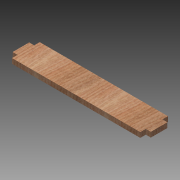
# Autodesk Inventor part: vigas
Saved by Autodesk Inventor 2016 (Build 200138000, 138)
## iProperties
Created: 2016-03-02
Part Number: vigas
Material: Wood (Birch)
Document SubType Name: Modeling
Designer: iberopuebla
Density: 0.55 g/cm^3
Appearance: Birch - Natural Polished
Author: iberopuebla
Autodesk Inventor part; units mm, degrees
ref_plane "YZ Plane" through (0, 0, 0) normal (1, 0, 0) x (0, 1, 0)
ref_plane "XZ Plane" through (0, 0, 0) normal (0, 1, 0) x (-1, 0, 0)
ref_plane "XY Plane" through (0, 0, 0) normal (0, 0, 1) x (1, 0, 0)
sketch "Sketch1" plane through (0, 0, 0) normal (0, 0, 1) x (1, 0, 0)
  line L0 (393.6245, -95.4118) -> (-70.3755, -95.4118)
  line L1 (-70.3755, 4.5882) -> (17.6245, 4.5882)
  line L2 (117.6245, 4.5882) -> (205.6245, 4.5882)
  line L3 (305.6245, 4.5882) -> (393.6245, 4.5882)
  line L4 (-88.3755, -15.4118) -> (-70.3755, -15.4118)
  line L5 (-70.3755, -75.4118) -> (-88.3755, -75.4118)
  line L6 (-88.3755, -75.4118) -> (-88.3755, -15.4118)
  line L7 (-70.3755, -95.4118) -> (-70.3755, -75.4118)
  line L8 (-70.3755, -15.4118) -> (-70.3755, 4.5882)
  line L9 (393.6245, -15.4118) -> (411.6245, -15.4118)
  line L10 (411.6245, -15.4118) -> (411.6245, -75.4118)
  line L11 (411.6245, -75.4118) -> (393.6245, -75.4118)
  line L12 (393.6245, 4.5882) -> (393.6245, -15.4118)
  line L13 (393.6245, -75.4118) -> (393.6245, -95.4118)
  line L14 (17.6245, 4.5882) -> (117.6245, 4.5882)
  line L15 (205.6245, 4.5882) -> (305.6245, 4.5882)
  point P0 (0, 0)
  dimension "d0" = 464
  dimension "d4" = 100
  dimension "d9" = 100
  dimension "d13" = 18
  dimension "d14" = 60
  dimension "d17" = 20
  dimension "d19" = 60
  dimension "d20" = 18
  dimension "d21" = 100
  constraints: 32 end point, 9 parallel, 7 perpendicular, 6 horizontal, 1 collinear
  measures "d0" distance of L0.start L0.end
  measures "d4" distance of L2.start L1.end
  measures "d9" distance of L3.start L2.end
  measures "d13" distance of L5.start L5.end
  measures "d14" distance of L4.end L5.start
  measures "d17" distance between parallel lines of L0 L5
  measures "d19" distance between parallel lines of L11 L9
  measures "d20" distance of L9.start L9.end
  measures "d21" distance between parallel lines of L0 L3
extrude "Extrusion1" add sketch "Sketch1" along normal blind 18
sketch "Sketch3" plane through (0, 0, 18) normal (0, 0, 1) x (1, 0, 0)
  line L0 (-70.3755, -15.4118) -> (-71.5069, -14.2805)
  line L1 (-70.3755, -15.4118) -> (-68.7755, -15.4118) construction
  line L2 (-70.3755, -75.4118) -> (-71.5069, -76.5432)
  line L3 (393.6245, -15.4118) -> (394.7558, -14.2805)
  line L4 (393.6245, -75.4118) -> (394.7558, -76.5432)
  circle A0 centre (-71.5069, -14.2805) radius 1.6
  circle A1 centre (-71.5069, -76.5432) radius 1.6
  circle A2 centre (394.7558, -14.2805) radius 1.6
  circle A3 centre (394.7558, -76.5432) radius 1.6
  point P0 (0, 0)
  dimension "d40" = 1.6
  dimension "d41" = 135
  dimension "d42" = 3.2
  dimension "d43" = 3.2
  dimension "d44" = 3.2
  dimension "d45" = 3.2
  constraints: 10 end point, 4 centre point, 4 coincident, 2 perpendicular, 1 equal length, 1 horizontal
  measures "d40" distance of L0.start L0.end
  measures "d41" angle of L1 L0
  measures "d42" diameter of A0
  measures "d43" diameter of A1
  measures "d44" diameter of A2
  measures "d45" diameter of A3
extrude "Extrusion3" cut sketch "Sketch3" against normal blind 20
body "Solid1"
